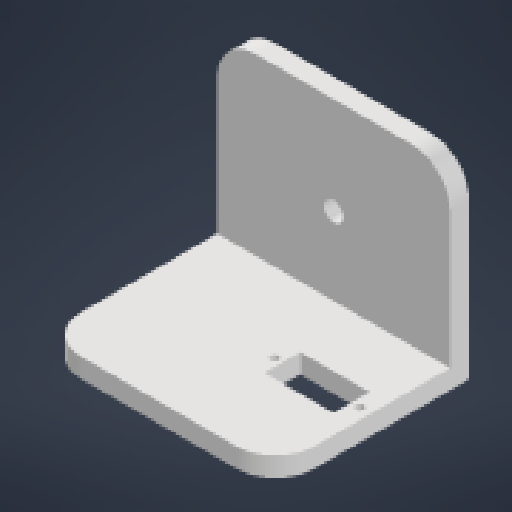
# Autodesk Inventor part: Base
Saved by Autodesk Inventor 2023 (Build 270158000, 158)
## iProperties
Created: 2022-11-05
Part Number: Base
Material: Generic
Document SubType Name: Modeling
Designer: cmzgt
Density: 1 g/cm^3
Appearance: Default
Author: cmzgt
Autodesk Inventor part; units mm, degrees
ref_plane "YZ Plane" through (0, 0, 0) normal (1, 0, 0) x (0, 1, 0)
ref_plane "XZ Plane" through (0, 0, 0) normal (0, 1, 0) x (-1, 0, 0)
ref_plane "XY Plane" through (0, 0, 0) normal (0, 0, 1) x (1, 0, 0)
sketch "Sketch1" plane through (0, 0, 0) normal (0, 0, 1) x (1, 0, 0)
  line L0 (38.1, -31.75) -> (-38.1, -31.75)
  line L1 (-38.1, -31.75) -> (-38.1, 31.75)
  line L2 (-38.1, 31.75) -> (38.1, 31.75)
  line L3 (38.1, 31.75) -> (38.1, -31.75)
  line L4 (38.1, -31.75) -> (-38.1, 31.75) construction
  line L5 (-38.1, -31.75) -> (38.1, 31.75) construction
  point P0 (0, 0)
  dimension "d0" = 76.2
  dimension "d1" = 63.5
  constraints: 12 end point, 2 midpoint, 2 parallel, 1 horizontal, 1 perpendicular
  measures "d0" distance of L1.end L2.end
  measures "d1" distance of L0.end L1.end
extrude "Extrusion1" add sketch "Sketch1" along normal blind 6.35
sketch "Sketch2" plane through (0, 0, 6.35) normal (0, 0, 1) x (1, 0, 0)
  line L0 (-38.1, -31.75) -> (38.1, -31.75) projected
  line L1 (38.1, -31.75) -> (38.1, 31.75) projected
  line L2 (-38.1, -31.75) -> (38.1, -31.75)
  line L3 (38.1, -31.75) -> (38.1, -25.4)
  line L4 (38.1, -25.4) -> (-38.1, -25.4)
  line L5 (-38.1, -25.4) -> (-38.1, -31.75)
  point P0 (0, 0)
  dimension "d4" = 6.35
  constraints: 8 end point, 2 parallel, 1 horizontal, 1 perpendicular, 1 point on line
  measures "d4" distance between parallel lines of L0 L4
extrude "Extrusion2" add sketch "Sketch2" along normal blind 57.15
fillet "Fillet1" radius 12.7 4 edges at (38.1, 31.75, 3.175) (-38.1, 31.75, 3.175) (38.1, -28.575, 63.5) (-38.1, -28.575, 63.5)
sketch "Sketch3" plane through (0, 0, 6.35) normal (0, 0, 1) x (1, 0, 0)
  circle A0 centre (0, 0) radius 3.175
  dimension "d8" = 6.35
  constraints: 1 centre point, 1 coincident
  measures "d8" diameter of A0
extrude "Extrusion3" cut sketch "Sketch3" against normal blind 25.4
sketch "Sketch4" plane through (-38.1, -25.4, 6.35) normal (0, 1, 0) x (1, 0, 0)
  line L0 (69.85, -20.2184) -> (69.85, -31.5468) projected
  line L1 (54.1906, -20.0152) -> (69.6468, -20.0152) projected
  line L2 (47.1932, -24.362) -> (47.1932, -20.2184) projected
  line L3 (47.1932, -31.5468) -> (47.1932, -27.4032) projected
  line L4 (69.6468, -31.75) -> (54.1906, -31.75) projected
  line L5 (51.7782, -31.75) -> (47.3964, -31.75) projected
  line L6 (69.85, -31.5468) -> (69.85, -31.75)
  line L7 (69.85, -31.75) -> (69.6468, -31.75)
  line L8 (69.6468, -31.75) -> (47.1932, -31.75)
  line L9 (47.1932, -31.75) -> (47.1932, -20.0152)
  line L10 (47.1932, -20.0152) -> (69.85, -20.0152)
  line L11 (69.85, -20.0152) -> (69.85, -31.5468)
  arc A0 (73.6332, -25.2857) -> (73.6332, -26.4795) centre (72.4408, -25.8826) ccw projected
  circle A1 centre (72.4408, -25.8826) radius 1.3335
  arc A2 (43.41, -26.4795) -> (43.41, -25.2857) centre (44.6024, -25.8826) ccw projected
  circle A3 centre (44.6024, -25.8826) radius 1.3335
  point P0 (38.1, 6.35)
  point P1 (47.1932, -27.4032)
  point P2 (73.6332, -25.2857)
  point P3 (43.41, -25.2857)
  dimension "d11" = 22.6568
  constraints: 12 end point, 4 perpendicular, 3 point on line, 2 centre point, 2 coincident, 2 concentric, 1 collinear, 1 vertical
  measures "d11" distance between parallel lines of L0 L9
extrude "Extrusion4" cut sketch "Sketch4" against normal blind 25.4
sketch "Sketch5" plane through (-38.1, -25.4, 6.35) normal (0, 1, 0) x (1, 0, 0)
  circle A0 centre (23.6728, -25.8826) radius 2.413
  circle A1 centre (52.9844, -25.8826) radius 2.413 projected
  line L0 (76.2, -25.8826) -> (0, -25.8826)
  circle A2 centre (23.6728, -25.8826) radius 0.8255
  circle A3 centre (52.9844, -25.8826) radius 0.8255 projected
  point P0 (38.1, 6.35)
  dimension "d14" = 4.826
  constraints: 2 centre point, 2 end point, 1 coincident, 1 equal radius, 1 horizontal, 1 point on line
  measures "d14" diameter of A0
ref_plane "Work Plane1" through (12.4714, -20.7772, 29.8196) normal (0, 1, 0) x (0, 0, 1)
extrude "Extrusion5" add sketch "Sketch5" along normal up to surface (4.6228 mm away) contours L0 A2 A0 | A0 L0 A2
body "Solid1"
